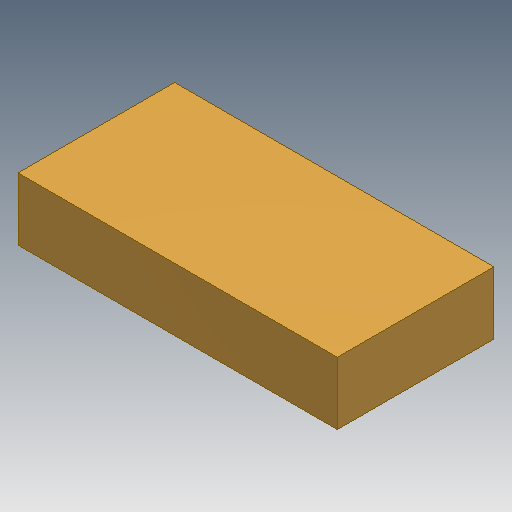
# Autodesk Inventor part: 10UF
Saved by Autodesk Inventor 2017 (Build 210142000, 142)
## iProperties
Part Number: 10UF
Material: Generisch
Document SubType Name: Modeling
Designer: Werkstatt
Density: 1 g/cm^3
Appearance: EIA3216, 10UF
Author: Werkstatt
Autodesk Inventor part; units mm, degrees
ref_plane "YZ Plane" through (0, 0, 0) normal (1, 0, 0) x (0, 1, 0)
ref_plane "XZ Plane" through (0, 0, 0) normal (0, 1, 0) x (-1, 0, 0)
ref_plane "XY Plane" through (0, 0, 0) normal (0, 0, 1) x (1, 0, 0)
sketch "EIA3216, 10UF_8" plane through (0, 0, 0) normal (0, 0, 1) x (1, 0, 0)
  line L0 (-2.6016, 1.2) -> (2.5, 1.2)
  line L1 (2.5, 1.2) -> (2.5, -1.3016)
  line L2 (2.5, -1.3016) -> (-2.6016, -1.3016)
  line L3 (-2.6016, -1.3016) -> (-2.6016, 1.2)
  constraints: 8 end point
extrude "Extrusion1" add sketch "EIA3216, 10UF_8" along normal blind 1
